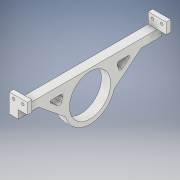
# Autodesk Inventor part: TubeBracket
Saved by Autodesk Inventor 2018 (Build 220112000, 112)
## iProperties
Created: 2019-04-15
Part Number: TubeBracket
Material: Generic
Document SubType Name: Modeling
Designer: anirudh
Density: 1 g/cm^3
Appearance: White
Mass: 49.1422 g
Surface Area: 187.719 cm^2
Volume: 49.1422 cm^3
Author: anirudh
Autodesk Inventor part; units mm, degrees
ref_plane "YZ Plane" through (0, 0, 0) normal (1, 0, 0) x (0, 1, 0)
ref_plane "XZ Plane" through (0, 0, 0) normal (0, 1, 0) x (-1, 0, 0)
ref_plane "XY Plane" through (0, 0, 0) normal (0, 0, 1) x (1, 0, 0)
sketch "Sketch1" plane through (0, 0, 0) normal (1, 0, 0) x (0, 1, 0)
  line L0 (32.385, 64.643) -> (43.575, 64.643)
  line L1 (43.575, 70.993) -> (21.075, 70.993)
  line L2 (21.075, 70.993) -> (-20.2641, 20.1469)
  line L3 (21.075, 19.297) -> (21.075, 58.7168)
  line L4 (21.075, 58.7168) -> (-3.618, 28.345)
  line L5 (32.385, -64.643) -> (43.575, -64.643)
  line L6 (43.575, -70.993) -> (21.075, -70.993)
  line L7 (21.075, -70.993) -> (-20.2641, -20.1469)
  line L8 (21.075, -19.297) -> (21.075, -58.7168)
  line L9 (21.075, -58.7168) -> (-3.618, -28.345)
  line L10 (43.575, 70.993) -> (47.385, 70.993)
  line L11 (47.385, 70.993) -> (47.385, 64.643)
  line L12 (47.385, 64.643) -> (43.575, 64.643)
  line L13 (32.385, 64.643) -> (32.385, -64.643)
  line L14 (47.385, -64.643) -> (43.575, -64.643)
  line L15 (47.385, -64.643) -> (47.385, -70.993)
  line L16 (47.385, -70.993) -> (43.575, -70.993)
  arc A0 (-3.618, 28.345) -> (-20.2641, 20.1469) centre (0, 0) ccw
  arc A1 (-20.2641, -20.1469) -> (-3.618, -28.345) centre (0, 0) ccw
  arc A2 (21.075, -19.297) -> (21.075, 19.297) centre (0, 0) ccw
  constraints: 34 end point, 6 point on circle, 4 perpendicular, 3 centre point, 2 parallel, 1 coincident, 1 point on line, 1 vertical
extrude "Extrusion1" add sketch "Sketch1" along normal blind 12.7
sketch "Sketch2" plane through (12.7, 0, 0) normal (1, 0, 0) x (0, 0, -1)
  line L0 (-28.345, -3.618) -> (-58.7168, 21.075) projected
  line L1 (-40.7634, 6.4785) -> (-34.8837, 1.6981)
  line L2 (-58.7168, 21.075) -> (-19.297, 21.075) projected
  line L3 (-35.489, 21.075) -> (-27.8496, 21.075)
  line L4 (19.297, 21.075) -> (58.7168, 21.075) projected
  line L5 (27.8496, 21.075) -> (35.489, 21.075)
  line L6 (58.7168, 21.075) -> (28.345, -3.618) projected
  line L7 (34.8837, 1.6981) -> (40.7634, 6.4785)
  arc A0 (-27.8496, 21.075) -> (-34.8837, 1.6981) centre (0, 0) ccw
  arc A1 (34.8837, 1.6981) -> (27.8496, 21.075) centre (0, 0) ccw
  arc A2 (-35.489, 21.075) -> (-40.7634, 6.4785) centre (0, 0) ccw
  arc A3 (40.7634, 6.4785) -> (35.489, 21.075) centre (0, 0) ccw
  point P0 (-51.7815, 15.4365)
  point P1 (-49.7786, 21.075)
  point P2 (-19.5423, 21.075)
  point P3 (19.5423, 21.075)
  point P4 (49.7786, 21.075)
  point P5 (51.7815, 15.4365)
  constraints: 8 end point, 8 point on circle, 8 point on line, 4 centre point, 2 coincident
extrude "Extrusion2" add sketch "Sketch2" against normal blind 12.7 contours L0 A2 L2 A0 | L4 A3 L6 A1
fillet "Fillet3" radius 3.175 8 edges at (6.35, 6.4785, -40.7634) (6.35, 21.075, -35.489) (6.35, 6.4785, 40.7634) (6.35, 21.075, 35.489) (6.35, 1.6981, -34.8837) (6.35, 21.075, -27.8496) (6.35, 21.075, 27.8496) (6.35, 1.6981, 34.8837)
sketch "Sketch3" plane through (0, 47.385, 70.993) normal (0, 0, 1) x (1, 0, 0)
  circle A0 centre (6.35, -7.5) radius 1.85
  point P0 (0, -47.385)
  point P1 (0, 0)
  dimension "d18" = 3.7
  constraints: 1 centre point
  measures "d18" diameter of A0
extrude "Extrusion3" cut sketch "Sketch3" against normal blind 150.8125
sketch "Sketch11" plane through (0, 47.385, 70.993) normal (0, 0, 1) x (1, 0, 0)
  line L0 (0, 0) -> (12.7, 0) projected
  line L1 (0, -15) -> (12.7, -15) projected
  line L2 (0, 0) -> (12.7, 0)
  line L3 (12.7, 0) -> (12.7, -15)
  line L4 (12.7, -15) -> (0, -15)
  line L5 (0, -15) -> (0, 0)
  point P0 (0, -47.385)
  constraints: 8 end point, 2 parallel, 1 horizontal, 1 perpendicular
extrude "Extrusion10" cut sketch "Sketch11" against normal blind 155.575
fillet "Fillet5" radius 1.905 2 edges at (6.35, 21.075, 58.7168) (6.35, 21.075, -58.7168)
sketch "Sketch13" plane through (0, 21.075, 70.993) normal (0, 0, 1) x (1, 0, 0)
  line L0 (0, 11.31) -> (0, 0) projected
  line L1 (12.7, 7.5) -> (12.7, 0) projected
  line L2 (0, 11.31) -> (12.7, 11.31)
  line L3 (12.7, 11.31) -> (12.7, 0.163)
  line L4 (12.7, 0.163) -> (0, 0.163)
  line L5 (0, 0.163) -> (0, 11.31)
  point P0 (0, -21.075)
  constraints: 8 end point, 2 parallel, 1 horizontal, 1 perpendicular
extrude "Extrusion11" add sketch "Sketch13" along normal blind 22.225
sketch "Sketch14" plane through (0, 21.075, -70.993) normal (0, 0, -1) x (-1, 0, 0)
  line L0 (-12.7, 0.163) -> (-12.7, 11.31) projected
  line L1 (-12.7, 11.31) -> (0, 11.31)
  line L2 (0, 11.31) -> (0, 0)
  line L3 (0, 0) -> (-12.7, 0)
  line L4 (-12.7, 0) -> (-12.7, 11.31)
  point P0 (0, -21.075)
  constraints: 8 end point, 2 parallel, 1 horizontal, 1 perpendicular
extrude "Extrusion12" add sketch "Sketch14" along normal blind 22.225
sketch "Sketch15" plane through (0, 32.385, 93.218) normal (0, 1, 0) x (1, 0, 0)
  line L0 (0, 0) -> (12.7, 0)
  line L1 (12.7, 0) -> (12.7, -6.35)
  line L2 (12.7, -6.35) -> (0, -6.35)
  line L3 (0, -6.35) -> (0, 0)
  line L4 (0, 186.436) -> (12.7, 186.436) projected
  line L5 (0, 186.436) -> (12.7, 186.436)
  line L6 (12.7, 186.436) -> (12.7, 192.786)
  line L7 (12.7, 192.786) -> (0, 192.786)
  line L8 (0, 192.786) -> (0, 186.436)
  point P0 (0, 93.218)
  dimension "d53" = 12.7
  dimension "d54" = 6.35
  dimension "d55" = 12.7
  dimension "d56" = 6.35
  constraints: 16 end point, 4 parallel, 2 horizontal, 2 perpendicular
  measures "d53" distance of L1.end L2.end
  measures "d54" distance of L0.end L1.end
  measures "d55" distance of L7.end L6.end
  measures "d56" distance of L6.end L5.end
extrude "Extrusion13" add sketch "Sketch15" along normal blind 15 and the other way blind 11.1506
sketch "Sketch16" plane through (0, 47.385, 99.568) normal (0, 0, 1) x (1, 0, 0)
  line L0 (0, 0) -> (0, -15) projected
  line L1 (0, 0) -> (12.7, 0)
  line L2 (12.7, 0) -> (12.7, -15)
  line L3 (12.7, -15) -> (0, -15)
  line L4 (0, -15) -> (0, 0)
  circle A0 centre (6.35, -5.214) radius 1.85
  point P0 (0, -47.385)
  dimension "d62" = 3.7
  constraints: 8 end point, 2 parallel, 1 centre point, 1 horizontal, 1 perpendicular
  measures "d62" diameter of A0
extrude "Extrusion14" cut sketch "Sketch16" against normal blind 227.8875 contours A0
sketch "Sketch17" plane through (0, 47.385, 99.568) normal (0, 0, 1) x (1, 0, 0)
  line L0 (12.7, 0) -> (0, 0) projected
  line L1 (0, 0) -> (-12.7, 0)
  line L2 (-12.7, 0) -> (-12.7, -15)
  line L3 (-12.7, -15) -> (0, -15)
  line L4 (0, -15) -> (0, 0)
  line L5 (12.7, 0) -> (12.7, -26.1506) projected
  line L6 (12.7, 0) -> (25.4, 0)
  line L7 (25.4, 0) -> (25.4, -15)
  line L8 (25.4, -15) -> (12.7, -15)
  line L9 (12.7, -15) -> (12.7, 0)
  circle A0 centre (6.35, -5.214) radius 1.85 projected
  circle A1 centre (-6.35, -5.214) radius 1.85
  circle A2 centre (19.05, -5.214) radius 1.85
  point P0 (0, -47.385)
  dimension "d65" = 12.7
  dimension "d66" = 15
  dimension "d67" = 12.7
  dimension "d68" = 3.7
  dimension "d69" = 3.7
  constraints: 16 end point, 4 parallel, 2 centre point, 2 horizontal, 2 perpendicular, 1 point on line
  measures "d65" distance of L3.end L2.end
  measures "d66" distance of L2.end L1.end
  measures "d67" distance of L7.end L8.end
  measures "d68" diameter of A1
  measures "d69" diameter of A2
extrude "Extrusion15" add sketch "Sketch17" against normal blind 6.35 contours L4 L3 L2 L1 | L6 L7 L8 L5
sketch "Sketch18" plane through (12.7, 47.385, -99.568) normal (0, 0, -1) x (-1, 0, 0)
  line L0 (-12.7, 0) -> (-12.7, -15) projected
  line L1 (-12.7, -15) -> (0, -15) projected
  line L2 (-12.7, 0) -> (0, 0)
  line L3 (0, 0) -> (0, -15)
  line L4 (0, -15) -> (-12.7, -15)
  line L5 (-12.7, -15) -> (-12.7, 0)
  line L6 (12.7, 0) -> (12.7, -15) projected
  line L7 (12.7, -15) -> (25.4, -15) projected
  line L8 (12.7, 0) -> (25.4, 0)
  line L9 (25.4, 0) -> (25.4, -15)
  line L10 (25.4, -15) -> (12.7, -15)
  line L11 (12.7, -15) -> (12.7, 0)
  circle A0 centre (-6.35, -5.214) radius 1.85 projected
  circle A1 centre (-6.35, -5.214) radius 1.85
  circle A2 centre (19.05, -5.214) radius 1.85 projected
  circle A3 centre (19.05, -5.214) radius 1.85
  point P0 (12.7, -47.385)
  constraints: 16 end point, 4 parallel, 2 centre point, 2 coincident, 2 horizontal, 2 perpendicular
extrude "Extrusion16" add sketch "Sketch18" against normal blind 6.35
sketch "Sketch19" plane through (12.7, 0, 0) normal (1, 0, 0) x (0, 0, -1)
  line L0 (-70.993, 21.075) -> (-70.993, 21.238) projected
  line L1 (-99.568, 32.385) -> (-99.568, 21.2344) projected
  line L2 (-70.993, 21.075) -> (-99.568, 21.075)
  line L3 (-99.568, 21.075) -> (-99.568, 21.2344)
  line L4 (-99.568, 21.2344) -> (-70.993, 21.2344)
  line L5 (-70.993, 21.2344) -> (-70.993, 21.075)
  point P0 (0, 0)
  point P1 (-99.568, 29.21)
  constraints: 8 end point, 2 parallel, 1 horizontal, 1 perpendicular
extrude "Extrusion17" add sketch "Sketch19" against normal blind 12.7
sketch "Sketch20" plane through (12.7, 0, 0) normal (1, 0, 0) x (0, 0, -1)
  line L0 (99.568, 21.2344) -> (93.218, 21.2344) projected
  line L1 (70.993, 21.075) -> (93.218, 21.075) projected
  line L2 (99.568, 21.2344) -> (93.218, 21.2344)
  line L3 (93.218, 21.2344) -> (93.218, 21.075)
  line L4 (93.218, 21.075) -> (99.568, 21.075)
  line L5 (99.568, 21.075) -> (99.568, 21.2344)
  point P0 (0, 0)
  constraints: 8 end point, 2 parallel, 1 horizontal, 1 perpendicular
extrude "Extrusion18" add sketch "Sketch20" against normal blind 12.7
sketch "Sketch21" plane through (-12.7, 32.385, 99.568) normal (0, -1, 0) x (1, 0, 0)
  line L0 (12.7, 0) -> (12.7, -6.35) projected
  line L1 (12.7, 0) -> (-22.745, 0)
  line L2 (-22.745, 0) -> (-22.745, -213.3172)
  line L3 (-22.745, -213.3172) -> (12.7, -213.3172)
  line L4 (12.7, -213.3172) -> (12.7, 0)
  point P0 (12.7, -99.568)
  constraints: 8 end point, 2 parallel, 1 horizontal, 1 perpendicular
extrude "Extrusion19" cut sketch "Sketch21" against normal blind 25.4
sketch "Sketch22" plane through (12.7, 0, 0) normal (1, 0, 0) x (0, 0, -1)
  line L0 (-70.993, 21.075) -> (-20.1469, -20.2641) projected
  circle A0 centre (0, 0) radius 28.575
  arc A1 (-28.8454, 19.69) -> (-34.7562, 3.4293) centre (0, 0) ccw projected
  arc A2 (-13.0755, 32.385) -> (13.0755, 32.385) centre (0, 0) ccw
  line L1 (93.218, 32.385) -> (-93.218, 32.385) projected
  line L2 (-13.0755, 32.385) -> (13.0755, 32.385)
  constraints: 3 point on circle, 2 coincident, 2 end point, 2 point on line, 1 centre point, 3 other
extrude "Extrusion20" add sketch "Sketch22" against normal blind 12.7
body "Solid1"
